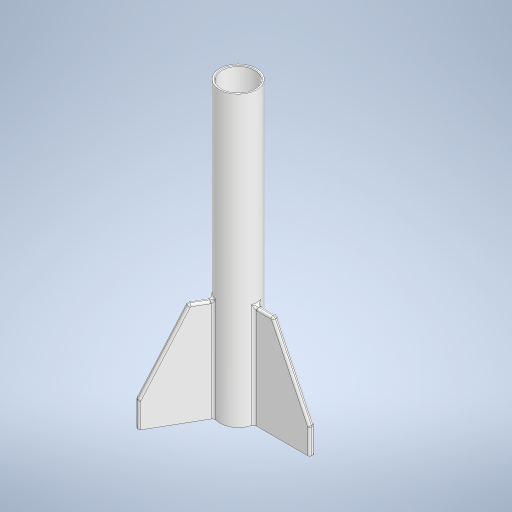
# Autodesk Inventor part: rocket_body
Saved by Autodesk Inventor 2024 (Build 280153000, 153)
## iProperties
Created: 2024-10-03
Part Number: rocket_body
Material: ABS Plastic
Document SubType Name: Modeling
Designer: soham
Density: 1.06 g/cm^3
Appearance: Smooth - White
Mass: 30.9964 g
Surface Area: 322.588 cm^2
Volume: 29.2419 cm^3
Author: soham
Autodesk Inventor part; units mm, degrees
ref_plane "YZ Plane" through (0, 0, 0) normal (1, 0, 0) x (0, 1, 0)
sketch "body_sketch" plane through (0, 0, 0) normal (0, 1, 0) x (-1, 0, 0)
  circle A0 centre (0, 0) radius 9.7
  circle A1 centre (0, 0) radius 10.9
  dimension "d0" = 19.4
  dimension "d1" = 21.8
  constraints: 2 centre point, 2 coincident
  measures "d0" diameter of A0
  measures "d1" diameter of A1
extrude "body_extrude" add sketch "body_sketch" along normal blind 170
fillet "body_top_fillet" radius 0.4 1 edges at (9.7, 170, 0)
sketch "fin_sketch" plane through (0, 0, 0) normal (0, 0, 1) x (1, 0, 0)
  line L0 (0, 0) -> (0, 60)
  line L1 (0, 60) -> (21.8, 60)
  line L2 (21.8, 60) -> (43.6, 15)
  line L3 (43.6, 15) -> (43.6, 0)
  line L4 (43.6, 0) -> (0, 0)
  line L5 (10.9, 0) -> (-10.9, 0) projected
  dimension "d24" = 60
  dimension "d25" = 43.6
  dimension "d26" = 21.8
  dimension "d27" = 15
  constraints: 10 end point, 1 collinear, 1 parallel, 1 perpendicular, 1 vertical
  measures "d24" distance of L0.start L0.end
  measures "d25" distance of L3.end L0.start
  measures "d26" distance of L0.end L1.end
  measures "d27" distance of L2.end L3.end
extrude "fin_extrude" add sketch "fin_sketch" along normal mid plane 3.2
fillet "fin_fillet" radius 1.6 5 edges at (10.7819, 30, 1.6) (10.7819, 30, -1.6) (10.9, 60, 0) (21.8, 60, 0) (43.6, 15, 0)
fillet "fin_leading_edge_fillet" radius 1.2 14 edges at (12.2396, 60.0077, 1.6) (11.0185, 60.6679, 2.0059) (21.6469, 59.7557, 1.6) (32.8386, 37.214, 1.6) (43.5595, 14.9907, 1.6) (43.6, 7.3164, 1.6) (16.5972, 60, 1.6) (43.5595, 14.9907, -1.6) (43.6, 7.3164, -1.6) (21.6469, 59.7557, -1.6) (16.5972, 60, -1.6) (12.2396, 60.0077, -1.6) (11.0185, 60.6679, -2.0059) (32.8386, 37.214, -1.6)
pattern_circular "fin_pattern" count 3 over 360 about axis through (0, -10, 0) along (0, 1, 0) of "fin_extrude", "fin_fillet", "fin_leading_edge_fillet"
sketch "fin_interior_cut_sketch" plane through (0, 0, 0) normal (0, 1, 0) x (-1, 0, 0)
  circle A0 centre (0, 0) radius 9.7
  dimension "d36" = 19.4
  constraints: 1 centre point, 1 coincident
  measures "d36" diameter of A0
extrude "fin_interior_cut" cut sketch "fin_interior_cut_sketch" along normal through all
ref_plane "Work Plane6" through (5.45, 0, -9.4397) normal (0.5, 0, -0.8660254) x (0, 1, 0)
ref_plane "Work Plane5" through (0, 0, 0) normal (0.5, 0, -0.8660254) x (0, 1, 0)
sketch "lug_sketch" plane through (5.45, 0, -9.4397) normal (0.5, 0, -0.8660254) x (0, 1, 0)
  line L0 (0, 0) -> (0, 3.5)
  line L1 (0, 7.7299) -> (61.6, 7.7299) projected
  line L2 (0, 3.5) -> (35, 3.5)
  line L3 (35, 3.5) -> (35, 0)
  line L4 (0, -7.7299) -> (0, 7.7299) projected
  line L5 (0, 0) -> (35, 0)
  line L6 (0, 0) -> (0, -3.5)
  line L7 (0, -3.5) -> (35, -3.5)
  line L8 (35, -3.5) -> (35, 0)
  line L9 (0, 2.7904) -> (0, 1.6) projected
  point P0 (0, 0)
  point P1 (0, 1.75)
  point P2 (0, 2.1952)
  dimension "d41" = 3.5
  dimension "d42" = 35
  constraints: 14 end point, 3 perpendicular, 2 midpoint, 2 symmetric about line, 1 horizontal, 1 point on line
  measures "d41" distance of L0.start L0.end
  measures "d42" distance of L0.end L2.end
extrude "lug_extrude" add sketch "lug_sketch" along normal blind 7 and the other way blind 0.8
sketch "lug_hole_sketch" plane through (8.1925, 35, -7.1898) normal (0, 1, 0) x (0.8660254, 0, 0.5)
  circle A0 centre (-3.5, 4.0772) radius 2.7
  line L0 (-7, 7.5772) -> (0, 7.5772) projected
  line L1 (0, 7.5772) -> (0, 0) projected
  point P0 (-3.5, -10.3228)
  dimension "d48" = 5.4
  dimension "d49" = 3.5
  dimension "d50" = 3.5
  constraints: 1 centre point
  measures "d48" diameter of A0
  measures "d49" distance from line of L0 A0.centre
  measures "d50" distance from line of L1 A0.centre
extrude "lug_hole_cut" cut sketch "lug_hole_sketch" against normal through all
fillet "lug_fillet" radius 3.5 5 edges at (8.1925, 17.5, -7.1898) (11.9811, 17.5, -13.7519) (5.9189, 17.5, -17.2519) (2.1303, 17.5, -10.6898) (5.45, 35, -9.4397)
sketch "bottom_hold_sketch" plane through (0, 0, 0) normal (0, 1, 0) x (-1, 0, 0)
  circle A0 centre (0, 0) radius 9.7 projected
  arc A1 (-9.6375, -1.0994) -> (-9.6375, 1.0994) centre (-10.8, 0) ccw
  line L0 (-56.8693, 0) -> (36.0157, 0) projected
  point P0 (-9.2, 0)
  dimension "d54" = 9.2
  dimension "d55" = 1.6
  constraints: 5 point on circle, 1 centre point, 1 point on line
  measures "d54" distance of point (-9.2, 0) A0.centre
  measures "d55" radius of A1
extrude "bottom_hold_extrude" add sketch "bottom_hold_sketch" along normal blind 2 contours A1 L0 A0 | A0 L0 A1 picked at (-9.5405, 0.2228) picked at (-9.5405, -0.2228)
sketch "top_hold_sketch" plane through (0, 0, 0) normal (1, 0, 0) x (0, 1, 0)
  line L0 (83.6, 9.7) -> (72, 9.7)
  line L1 (72, 9.7) -> (73.6, 8.1)
  line L2 (73.6, 8.1) -> (83.6, 8.1)
  line L3 (83.6, 8.1) -> (83.6, 9.7)
  line L4 (0, 53.3673) -> (0, -53.3673) projected
  line L5 (-34, 0) -> (204, 0) projected
  point P0 (0, 0)
  point P1 (77.8, 9.7)
  dimension "d74" = 72
  dimension "d75" = 45
  dimension "d76" = 9.7
  dimension "d77" = 1.6
  dimension "d78" = 11.6
  constraints: 8 end point, 1 horizontal, 1 midpoint, 1 parallel, 1 perpendicular
  measures "d74" distance from line of L4 L0.end
  measures "d75" angle of L1 L0
  measures "d76" distance from line of L5 point (77.8, 9.7)
  measures "d77" distance of L2.end L0.start
  measures "d78" distance of L0.start L0.end
revolve "top_hold_revolve" add sketch "top_hold_sketch" angle 360 about axis through (0, 0, 0) along (0, 1, 0)
ref_plane "Work Plane10" through (0, 140, 0) normal (0, 1, 0) x (-1, 0, 0)
sketch "cord_attachment_sketch" plane through (0, 0, 0) normal (0, 0, 1) x (1, 0, 0)
  line L0 (3.1, 135) -> (9.7, 135)
  line L1 (9.7, 135) -> (9.7, 127.6)
  line L2 (9.7, 127.6) -> (3.1, 134.2)
  line L3 (3.1, 134.2) -> (3.1, 135)
  line L4 (-36.0157, 0) -> (56.8693, 0) projected
  line L5 (0, 204) -> (0, -34) projected
  point P0 (0, 0)
  point P1 (6.4, 135)
  point P2 (3.1, 134.6)
  dimension "d81" = 6.6
  dimension "d82" = 7.4
  dimension "d83" = 45
  dimension "d84" = 135
  dimension "d85" = 3.1
  constraints: 8 end point, 2 midpoint, 1 horizontal, 1 parallel, 1 perpendicular
  measures "d81" distance of L0.start L0.end
  measures "d82" distance of L0.end L1.end
  measures "d83" angle of L2 L1
  measures "d84" distance from line of L4 point (6.4, 135)
  measures "d85" distance from line of point (3.1, 134.6) L5
extrude "cord_attachment_extrude" add sketch "cord_attachment_sketch" along normal mid plane 6.6
sketch "attachment_hole_sketch" plane through (3.1, 135, -3.3) normal (0, 1, 0) x (1, 0, 0)
  circle A0 centre (3.3, -3.3) radius 2.5
  line L0 (0, 0) -> (0, -6.6) projected
  line L1 (6.0214, -6.6) -> (0, -6.6) projected
  point P0 (-3.1, -3.3)
  dimension "d88" = 5
  dimension "d89" = 3.3
  dimension "d90" = 3.3
  constraints: 1 centre point
  measures "d88" diameter of A0
  measures "d89" distance from line of L0 A0.centre
  measures "d90" distance from line of L1 A0.centre
extrude "attachment_hole_cut" cut sketch "attachment_hole_sketch" against normal up to next
equation "\"d0\" = interior_diameter"
equation "\"d1\" = exterior_diameter"
equation "\"d25\" = 2 * exterior_diameter"
equation "\"d26\" = exterior_diameter"
equation "\"d36\" = interior_diameter"
equation "\"d76\" = 0.5 * interior_diameter"
equation "\"interior_diameter\" = 19.4"
equation "\"exterior_diameter\" = interior_diameter + 2 * wall_thickness"
equation "\"wall_thickness\" = 1.2"
equation "\"d40\" = 0.5 * exterior_diameter"
